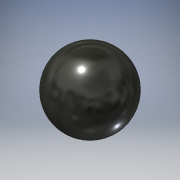
# Autodesk Inventor part: Tank
Saved by Autodesk Inventor 2017.2 (Build 212233000, 233)
## iProperties
Created: 2017-03-31
Part Number: Tank
Material: Generic
Document SubType Name: Modeling
Designer: haden
Density: 1 g/cm^3
Appearance: Carbon Fiber 1
Author: haden
Autodesk Inventor part; units mm, degrees
ref_plane "YZ Plane" through (0, 0, 0) normal (1, 0, 0) x (0, 1, 0)
ref_plane "XZ Plane" through (0, 0, 0) normal (0, 1, 0) x (-1, 0, 0)
sketch "Sketch1" plane through (0, 0, 0) normal (0, 0, 1) x (1, 0, 0)
  arc A0 (0, -56300) -> (0, 56300) centre (0, 0) ccw
  arc A1 (0, -57000) -> (0, 57000) centre (0, 0) ccw
  line L0 (0, 57000) -> (0, 56300)
  line L1 (0, -57000) -> (0, -56300)
  dimension "d1" = 56300
  dimension "d2" = 700
  constraints: 4 end point, 4 point on circle, 2 centre point, 2 coincident, 2 point on line, 1 collinear, 1 vertical
  measures "d1" distance of L0.end point (0, 0)
  measures "d2" radial gap between concentric circles of A1 A0
revolve "Revolution1" add sketch "Sketch1" angle 360 about axis through (0, 57000, 0) along (0, -1, 0)
ref_plane "Work Plane1" through (0, 0, 57000) normal (0, 0, 1) x (1, 0, 0)
sketch "Sketch2" plane through (0, 0, 57000) normal (0, 0, 1) x (1, 0, 0)
  circle A0 centre (0, 0) radius 500
  circle A1 centre (0, 0) radius 57000 projected
  dimension "d4" = 1000
  constraints: 1 centre point, 1 concentric
  measures "d4" diameter of A0
extrude "Extrusion1" cut sketch "Sketch2" against normal blind 5000 contours A0
body "Solid1"
